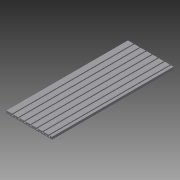
# Autodesk Inventor part: ISEL T-SLOT Table Section
Saved by Autodesk Inventor 2013 (Build 170138000, 138)
## iProperties
Created: 2016-08-23
Part Number: ISEL T-SLOT Table Section
Material: Generic
Document SubType Name: Modeling
Designer: Jonathan White
Density: 1 g/cm^3
Author: Jonathan White
Autodesk Inventor part; units mm, degrees
ref_plane "YZ Plane" through (0, 0, 0) normal (1, 0, 0) x (0, 1, 0)
ref_plane "XZ Plane" through (0, 0, 0) normal (0, 1, 0) x (-1, 0, 0)
ref_plane "XY Plane" through (0, 0, 0) normal (0, 0, 1) x (1, 0, 0)
sketch "Sketch1" plane through (0, 0, 0) normal (0, 0, 1) x (1, 0, 0)
  line L0 (375.0056, 0) -> (396.0038, 0)
  line L1 (750.0112, 0) -> (750.0112, 20)
  line L2 (750.0112, 20) -> (729.0054, 20)
  line L3 (375.0056, 20) -> (375.0056, 0)
  line L4 (750.0036, 20) -> (750.0036, 0)
  line L5 (392.7526, 5.0038) -> (396.0038, 5.0038)
  line L6 (404.0048, 5.0038) -> (407.256, 5.0038)
  line L7 (407.256, 5.0038) -> (407.256, 12.0142)
  line L8 (407.256, 12.0142) -> (392.7526, 12.0142)
  line L9 (392.7526, 12.0142) -> (392.7526, 5.0038)
  line L10 (404.0048, 5.0038) -> (404.0048, 0)
  line L11 (396.0038, 5.0038) -> (396.0038, 0)
  line L12 (442.7525, 5.0038) -> (446.0037, 5.0038)
  line L13 (454.0047, 5.0038) -> (457.2559, 5.0038)
  line L14 (457.2559, 5.0038) -> (457.2559, 12.0142)
  line L15 (457.2559, 12.0142) -> (442.7525, 12.0142)
  line L16 (442.7525, 12.0142) -> (442.7525, 5.0038)
  line L17 (454.0047, 5.0038) -> (454.0047, 0)
  line L18 (446.0037, 5.0038) -> (446.0037, 0)
  line L19 (492.7524, 5.0038) -> (496.0036, 5.0038)
  line L20 (504.0046, 5.0038) -> (507.2558, 5.0038)
  line L21 (507.2558, 5.0038) -> (507.2558, 12.0142)
  line L22 (507.2558, 12.0142) -> (492.7524, 12.0142)
  line L23 (492.7524, 12.0142) -> (492.7524, 5.0038)
  line L24 (504.0046, 5.0038) -> (504.0046, 0)
  line L25 (496.0036, 5.0038) -> (496.0036, 0)
  line L26 (542.7523, 5.0038) -> (546.0035, 5.0038)
  line L27 (554.0045, 5.0038) -> (557.2557, 5.0038)
  line L28 (557.2557, 5.0038) -> (557.2557, 12.0142)
  line L29 (557.2557, 12.0142) -> (542.7523, 12.0142)
  line L30 (542.7523, 12.0142) -> (542.7523, 5.0038)
  line L31 (554.0045, 5.0038) -> (554.0045, 0)
  line L32 (546.0035, 5.0038) -> (546.0035, 0)
  line L33 (592.7522, 5.0038) -> (596.0034, 5.0038)
  line L34 (604.0044, 5.0038) -> (607.2556, 5.0038)
  line L35 (607.2556, 5.0038) -> (607.2556, 12.0142)
  line L36 (607.2556, 12.0142) -> (592.7522, 12.0142)
  line L37 (592.7522, 12.0142) -> (592.7522, 5.0038)
  line L38 (604.0044, 5.0038) -> (604.0044, 0)
  line L39 (596.0034, 5.0038) -> (596.0034, 0)
  line L40 (642.7521, 5.0038) -> (646.0033, 5.0038)
  line L41 (654.0043, 5.0038) -> (657.2555, 5.0038)
  line L42 (657.2555, 5.0038) -> (657.2555, 12.0142)
  line L43 (657.2555, 12.0142) -> (642.7521, 12.0142)
  line L44 (642.7521, 12.0142) -> (642.7521, 5.0038)
  line L45 (654.0043, 5.0038) -> (654.0043, 0)
  line L46 (646.0033, 5.0038) -> (646.0033, 0)
  line L47 (692.752, 5.0038) -> (696.0032, 5.0038)
  line L48 (704.0042, 5.0038) -> (707.2554, 5.0038)
  line L49 (707.2554, 5.0038) -> (707.2554, 12.0142)
  line L50 (707.2554, 12.0142) -> (692.752, 12.0142)
  line L51 (692.752, 12.0142) -> (692.752, 5.0038)
  line L52 (704.0042, 5.0038) -> (704.0042, 0)
  line L53 (696.0032, 5.0038) -> (696.0032, 0)
  line L54 (432.2572, 14.9962) -> (429.006, 14.9962)
  line L55 (421.005, 14.9962) -> (417.7538, 14.9962)
  line L56 (417.7538, 14.9962) -> (417.7538, 7.9858)
  line L57 (417.7538, 7.9858) -> (432.2572, 7.9858)
  line L58 (432.2572, 7.9858) -> (432.2572, 14.9962)
  line L59 (421.005, 14.9962) -> (421.005, 20)
  line L60 (429.006, 14.9962) -> (429.006, 20)
  line L61 (482.2571, 14.9962) -> (479.0059, 14.9962)
  line L62 (471.0049, 14.9962) -> (467.7537, 14.9962)
  line L63 (467.7537, 14.9962) -> (467.7537, 7.9858)
  line L64 (467.7537, 7.9858) -> (482.2571, 7.9858)
  line L65 (482.2571, 7.9858) -> (482.2571, 14.9962)
  line L66 (471.0049, 14.9962) -> (471.0049, 20)
  line L67 (479.0059, 14.9962) -> (479.0059, 20)
  line L68 (532.257, 14.9962) -> (529.0058, 14.9962)
  line L69 (521.0048, 14.9962) -> (517.7536, 14.9962)
  line L70 (517.7536, 14.9962) -> (517.7536, 7.9858)
  line L71 (517.7536, 7.9858) -> (532.257, 7.9858)
  line L72 (532.257, 7.9858) -> (532.257, 14.9962)
  line L73 (521.0048, 14.9962) -> (521.0048, 20)
  line L74 (529.0058, 14.9962) -> (529.0058, 20)
  line L75 (582.2569, 14.9962) -> (579.0057, 14.9962)
  line L76 (571.0047, 14.9962) -> (567.7535, 14.9962)
  line L77 (567.7535, 14.9962) -> (567.7535, 7.9858)
  line L78 (567.7535, 7.9858) -> (582.2569, 7.9858)
  line L79 (582.2569, 7.9858) -> (582.2569, 14.9962)
  line L80 (571.0047, 14.9962) -> (571.0047, 20)
  line L81 (579.0057, 14.9962) -> (579.0057, 20)
  line L82 (632.2568, 14.9962) -> (629.0056, 14.9962)
  line L83 (621.0046, 14.9962) -> (617.7534, 14.9962)
  line L84 (617.7534, 14.9962) -> (617.7534, 7.9858)
  line L85 (617.7534, 7.9858) -> (632.2568, 7.9858)
  line L86 (632.2568, 7.9858) -> (632.2568, 14.9962)
  line L87 (621.0046, 14.9962) -> (621.0046, 20)
  line L88 (629.0056, 14.9962) -> (629.0056, 20)
  line L89 (682.2567, 14.9962) -> (679.0055, 14.9962)
  line L90 (671.0045, 14.9962) -> (667.7533, 14.9962)
  line L91 (667.7533, 14.9962) -> (667.7533, 7.9858)
  line L92 (667.7533, 7.9858) -> (682.2567, 7.9858)
  line L93 (682.2567, 7.9858) -> (682.2567, 14.9962)
  line L94 (671.0045, 14.9962) -> (671.0045, 20)
  line L95 (679.0055, 14.9962) -> (679.0055, 20)
  line L96 (732.2566, 14.9962) -> (729.0054, 14.9962)
  line L97 (721.0044, 14.9962) -> (717.7532, 14.9962)
  line L98 (717.7532, 14.9962) -> (717.7532, 7.9858)
  line L99 (717.7532, 7.9858) -> (732.2566, 7.9858)
  line L100 (732.2566, 7.9858) -> (732.2566, 14.9962)
  line L101 (721.0044, 14.9962) -> (721.0044, 20)
  line L102 (729.0054, 14.9962) -> (729.0054, 20)
  line L103 (404.0048, 0) -> (446.0037, 0)
  line L104 (454.0047, 0) -> (496.0036, 0)
  line L105 (504.0046, 0) -> (546.0035, 0)
  line L106 (554.0045, 0) -> (596.0034, 0)
  line L107 (604.0044, 0) -> (646.0033, 0)
  line L108 (621.0046, 20) -> (579.0057, 20)
  line L109 (654.0043, 0) -> (696.0032, 0)
  line L110 (671.0045, 20) -> (629.0056, 20)
  line L111 (704.0042, 0) -> (750.0112, 0)
  line L112 (721.0044, 20) -> (679.0055, 20)
  line L113 (571.0047, 20) -> (529.0058, 20)
  line L114 (521.0048, 20) -> (479.0059, 20)
  line L115 (471.0049, 20) -> (429.006, 20)
  line L116 (421.005, 20) -> (375.0056, 20)
  point P0 (0, 0)
  constraints: 234 end point
extrude "Extrusion1" add sketch "Sketch1" against normal blind 999.998
body "Solid1"
